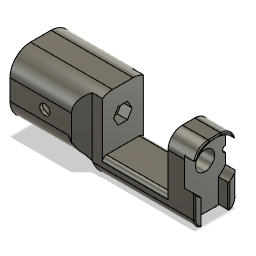
Overall_Assembly2 v12 (Autodesk Fusion 360 archive; units mm, degrees)
design "ElbowFork_4"
Autodesk Fusion 360 part; units mm, degrees
sketch "Sketch1" plane through (0, 0, 0) normal (0, 1, 0) x (1, 0, 0)
  line L0 (-40, 15) -> (-10, 15)
  line L1 (-10, 15) -> (-10, -15)
  line L2 (-40, -15) -> (-10, -15)
  line L3 (-10, -15) -> (-6.6882, -19.9677)
  line L4 (-5, 0) -> (-5, 15)
  line L5 (27, 0) -> (27, 15)
  line L6 (-5, 0) -> (-5, -10)
  line L7 (-5, -10) -> (27, -10)
  line L8 (27, -10) -> (27, 0)
  line L9 (30, -19.9677) -> (-6.6882, -19.9677)
  line L10 (30, 15) -> (40, 15)
  line L11 (40, 15) -> (40, -19.9677)
  line L12 (40, -19.9677) -> (30, -19.9677)
  line L13 (-10, 15) -> (-5, 15)
  line L14 (27, 15) -> (30, 15)
  line L15 (27, 15) -> (30, 15)
  line L16 (-40, 0) -> (-40, 15)
  line L17 (-40, 0) -> (-40, -15)
  constraint perpendicular L1 L2
  constraint perpendicular L4 L13
  constraint coincident L5.end L13
  constraint parallel L4 L6
  constraint perpendicular L4 L7
  constraint perpendicular L7 L8
  constraint collinear L13 L14
  constraint perpendicular L0 L16
  constraint perpendicular L2 L17
extrude "Extrude1" add sketch "Sketch1" along normal blind 30 makes body 1
sketch "Sketch2" plane through (-40, 0, 0) normal (-1, 0, 0) x (0, 0, 1)
  line L0 (-15, 0) -> (15, 0)
  line L1 (15, 0) -> (15, 30)
  line L2 (15, 30) -> (-15, 30)
  line L3 (-15, 30) -> (-15, 0)
  line L4 (-15, 0) -> (15, 0)
  line L5 (15, 0) -> (15, 30)
  line L6 (15, 30) -> (-15, 30)
  line L7 (-15, 30) -> (-15, 0)
  circle A0 centre (0, 15) radius 13.6
  point P0 (0, 15)
  dimension "d37" = 27.2
  constraint coincident P0 A0.centre
  measures "d37" diameter of A0
extrude "Extrude2" cut sketch "Sketch2" against normal blind 22 contours A0 bodies 1
sketch "Sketch3" plane through (0, 30, 0) normal (0, 1, 0) x (-1, 0, 0)
  line L0 (40, -15) -> (40, 15)
  line L1 (40, 15) -> (10, 15)
  line L2 (10, 15) -> (6.6882, 19.9677)
  line L3 (6.6882, 19.9677) -> (-40, 19.9677)
  line L4 (-40, 19.9677) -> (-40, -15)
  line L5 (-40, -15) -> (-27, -15)
  line L6 (-27, -15) -> (-27, 10)
  line L7 (-27, 10) -> (5, 10)
  line L8 (5, 10) -> (5, -15)
  line L9 (5, -15) -> (40, -15)
  line L10 (10, 15) -> (10, -15)
  constraint coincident L1.end L2.start
  constraint coincident L9 L10.end
  constraint perpendicular L9 L10
extrude "Extrude3" cut sketch "Sketch3" against normal blind 5 contours L2 L3 L4 L5 L6 L7 L8 L9 L10 bodies 1
extrude "Extrude4" cut sketch "Sketch1" along normal blind 5 contours L1 L3 L4 L5 L6 L7 L8 L9 L10 L11 L12 L13 L14 L15 bodies 1
chamfer "Chamfer1" distance 5 angle 45 2 edges at (-10, 30, 0) (-10, 0, 0) on bodies 1
fillet "Fillet1" radius 10 4 edges at (-27.5, 30, -15) (-27.5, 30, 15) (-27.5, 0, -15) (-27.5, 0, 15) on bodies 1
sketch "Sketch4" plane through (40, 0, 0) normal (1, 0, 0) x (0, 0, -1)
  line L0 (-19.9677, 5) -> (15, 5)
  line L1 (15, 5) -> (15, 25)
  line L2 (15, 25) -> (-19.9677, 25)
  line L3 (-19.9677, 25) -> (-19.9677, 5)
  line L4 (2.5, 15) -> (2.5, 5) construction
  circle A0 centre (2.5, 5) radius 1.5
  line L5 (-25, 14.9495) -> (-25, 21.4495)
  line L6 (-25, 14.9495) -> (-25, 8.4495)
  line L7 (-25, 21.4495) -> (-7.6195, 21.4495)
  line L8 (-25, 8.4495) -> (-7.5544, 8.4495)
  arc A1 (-7.5544, 8.4495) -> (-7.6195, 21.4495) centre (2.5, 15) ccw
  circle A2 centre (2.5, 15) radius 4.65
  dimension "d38" = 3
  dimension "d39" = 24
  dimension "d40" = 6.5
  dimension "d41" = 6.5
  dimension "d46" = 9.3
  constraint coincident L0 L4.end
  constraint perpendicular L0 L4
  constraint coincident L4.end A0.centre
  constraint perpendicular L5 L7
  constraint perpendicular L6 L8
  constraint concentric A1 A2
  measures "d38" diameter of A0
  measures "d39" diameter of A1
  measures "d40" distance of L5.start L5.end
  measures "d41" distance of L5.start L6.end
  measures "d46" diameter of A2
extrude "Extrude5" cut sketch "Sketch4" against normal blind 5 contours L0 L2 L3 A0 L7 L8 A1 | A2 bodies 1
extrude "Extrude6" cut sketch "Sketch4" against normal blind 16 contours A2 bodies 1
fillet "Fillet2" radius 2 2 edges at (11, 25, 10) (11, 5, 10) on bodies 1
sketch "Sketch5" plane through (-5, 0, 0) normal (1, 0, 0) x (0, 0, -1)
  arc A0 (13.6603, 5) -> (15, 10) centre (5, 10) ccw
  line L0 (15, 10) -> (15, 20)
  arc A1 (15, 20) -> (13.6603, 25) centre (5, 20) ccw
  line L1 (13.6603, 25) -> (-12, 25)
  arc A2 (-10, 23) -> (-12, 25) centre (-12, 23) ccw
  line L2 (-10, 23) -> (-10, 7)
  arc A3 (-12, 5) -> (-10, 7) centre (-12, 7) ccw
  line L3 (-12, 5) -> (13.6603, 5)
  line L4 (4.45, 11.6225) -> (2.5, 10.4967)
  line L5 (-1.4, 15) -> (-1.4, 17.2517)
  line L6 (0.55, 18.3775) -> (-1.4, 17.2517)
  line L7 (4.45, 18.3775) -> (6.4, 17.2517)
  line L8 (4.45, 18.3775) -> (2.5, 19.5033)
  line L9 (0.55, 18.3775) -> (2.5, 19.5033)
  line L10 (0.55, 11.6225) -> (-1.4, 12.7483)
  line L11 (4.45, 11.6225) -> (6.4, 12.7483)
  line L12 (6.4, 15) -> (6.4, 17.2517)
  line L13 (-1.4, 15) -> (-1.4, 12.7483)
  line L14 (0.55, 11.6225) -> (2.5, 10.4967)
  line L15 (6.4, 15) -> (6.4, 12.7483)
  circle A4 centre (2.5, 15) radius 2.5
  dimension "d36" = 5
  measures "d36" diameter of A4
extrude "Extrude9" cut sketch "Sketch5" against normal blind 5 contours L4 L5 L6 L7 L8 L9 L10 L11 L12 L13 L14 L15 | A4 bodies 1
extrude "Extrude8" cut sketch "Sketch5" against normal blind 15 contours A4 bodies 1
fillet "Fillet3" radius 7 2 edges at (33.5, 25, -15) (33.5, 5, -15) on bodies 1
fillet "Fillet4" radius 4.5 2 edges at (16.6559, 25, 19.9677) (16.6559, 5, 19.9677) on bodies 1
sketch "Sketch6" plane through (0, 30, 0) normal (0, 1, 0) x (-1, 0, 0)
  line L0 (40, 5) -> (16.6667, 5)
  line L1 (16.6667, 5) -> (15, 7.5)
  line L2 (15, 7.5) -> (15, -5)
  line L3 (15, -5) -> (40, -5)
  line L4 (40, -5) -> (40, 5)
  circle A0 centre (28, 0) radius 2.5
  dimension "d33" = 5
  measures "d33" diameter of A0
extrude "Extrude10" cut sketch "Sketch6" against normal blind 58 contours A0 bodies 1
copy_body "Body->Comp1" bodies 1 removing the originals makes body 2 in component "Component"
extrude "Extrude1'" cut 1 faces at (40, 5.54, -2.6771) along direction (-1, 0, 0) blind 9 on bodies 2 bodies 2 in component "Component"
fillet "Fillet1'" radius 0.5 14 edges at (40, 25, 9.8005) (40, 24.0016, 18.2941) (40, 5.9661, 18.2536) (40, 5, 9.8005) (40, 22.4594, -13.3958) (40, 15, -15) (40, 7.5406, -13.3958) (40, 21.4495, 13.7429) (40, 8.4495, 13.6989) (37.5, 21.4495, 19.8664) (37.5, 8.4495, 19.8434) (35, 8.9711, 19.9365) (35, 15, 19.9677) (35, 20.9775, 19.9423) on bodies 2 in component "Component"
move_face "OffsetFaces1" offset 5 1 faces at (-40, 4.1882, 10.0012) on bodies 2 in component "Component"
move_face "OffsetFaces2" offset -1 1 faces at (5.6667, 12.3333, 10) on bodies 2 in component "Component"
component "Component" placed x (1, 0, 0) y (0, 1, 0) z (0, 0, 1) at (0, 0, 0)

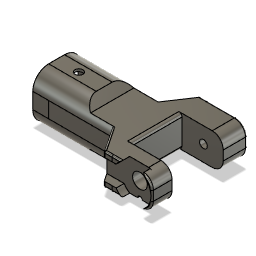
design "SholderFork_1"
Autodesk Fusion 360 part; units mm, degrees
sketch "Sketch1" plane through (0, 0, 0) normal (0, 1, 0) x (1, 0, 0)
  line L0 (-50, -15) -> (-10, -15)
  line L1 (-50, 15) -> (-10, 15)
  line L2 (5, -15) -> (5, 15)
  line L3 (30, 30) -> (5, 30)
  line L4 (30, -30) -> (5, -30)
  line L5 (5, -15) -> (30, -15)
  line L6 (30, -15) -> (30, -30)
  line L7 (5, 15) -> (30, 15)
  line L8 (30, 15) -> (30, 30)
  line L9 (-10, -15) -> (0, -30)
  line L10 (0, -30) -> (5, -30)
  line L11 (-10, 15) -> (0, 30)
  line L12 (0, 30) -> (5, 30)
  line L13 (-10, 15) -> (-10, -15)
  line L14 (-50, 15) -> (-60, 15)
  line L15 (-60, 15) -> (-60, -15)
  line L16 (-60, -15) -> (-50, -15)
  constraint horizontal L3
  constraint perpendicular L2 L5
  constraint perpendicular L4 L6
  constraint perpendicular L2 L7
  constraint perpendicular L3 L8
  constraint perpendicular L0 L13
  constraint perpendicular L14 L15
extrude "Extrude1" add sketch "Sketch1" along normal blind 30 makes body 1
sketch "Sketch3" plane through (-60, 0, 0) normal (-1, 0, 0) x (0, 0, 1)
  line L0 (-15, 0) -> (15, 0)
  line L1 (15, 0) -> (15, 30)
  line L2 (15, 30) -> (-15, 30)
  line L3 (-15, 30) -> (-15, 0)
  circle A0 through (13.6, 15, 10) (-6.8, 26.7779, 10) (-6.8, 3.2221, 10)
  line L4 (-15, 0) -> (15, 0)
  line L5 (15, 0) -> (15, 30)
  line L6 (15, 30) -> (-15, 30)
  line L7 (-15, 30) -> (-15, 0)
  dimension "d64" = 27.2
extrude "Extrude3" cut sketch "Sketch3" against normal blind 36 contours A0 in plane through (-70, 0, 0) normal (-1, 0, 0) bodies 1
sketch "Sketch4" plane through (0, 30, 0) normal (0, 1, 0) x (-1, 0, 0)
  line L0 (50, 15) -> (10, 15)
  line L1 (10, 15) -> (0, 30)
  line L2 (0, 30) -> (-5, 30)
  line L3 (-5, 30) -> (-30, 30)
  line L4 (-30, 30) -> (-30, 15)
  line L5 (-30, 15) -> (-5, 15)
  line L6 (-5, 15) -> (-5, -15)
  line L7 (-5, -15) -> (-30, -15)
  line L8 (-30, -15) -> (-30, -30)
  line L9 (-30, -30) -> (-5, -30)
  line L10 (-5, -30) -> (0, -30)
  line L11 (0, -30) -> (10, -15)
  line L12 (10, -15) -> (60, -15)
  line L13 (25, -10) -> (25, -15)
  line L14 (25, -10) -> (25, 15)
  line L15 (60, -15) -> (60, 15)
  line L16 (60, 15) -> (50, 15)
  constraint coincident L12 L13.end
  constraint perpendicular L12 L13
  constraint coincident L0 L14.end
  constraint perpendicular L0 L14
extrude "Extrude4" cut sketch "Sketch4" against normal blind 5 contours L0 L1 L2 L3 L4 L5 L6 L7 L8 L9 L10 L11 L12 L13 L14 bodies 1
sketch "Sketch5" plane through (0, 0, 0) normal (0, -1, 0) x (1, 0, 0)
  line L0 (-60, -15) -> (-10, -15)
  line L1 (-10, -15) -> (0, -30)
  line L2 (0, -30) -> (5, -30)
  line L3 (5, -30) -> (30, -30)
  line L4 (30, -30) -> (30, -15)
  line L5 (30, -15) -> (5, -15)
  line L6 (5, -15) -> (5, 15)
  line L7 (5, 15) -> (30, 15)
  line L8 (30, 15) -> (30, 30)
  line L9 (30, 30) -> (5, 30)
  line L10 (5, 30) -> (0, 30)
  line L11 (0, 30) -> (-10, 15)
  line L12 (-10, 15) -> (-50, 15)
  line L13 (-25, 14) -> (-25, 15)
  line L14 (-25, 14) -> (-25, -15)
  line L15 (-50, 15) -> (-60, 15)
  line L16 (-60, 15) -> (-60, -15)
  constraint coincident L12 L13.end
  constraint perpendicular L12 L13
  constraint perpendicular L12 L14
extrude "Extrude5" cut sketch "Sketch5" against normal blind 5 contours L0 L1 L2 L3 L4 L5 L6 L7 L8 L9 L10 L11 L12 L13 L14 bodies 1
chamfer "Chamfer1" distance 5 angle 45 2 edges at (-25, 0, 0) (-25, 30, 0) on bodies 1
fillet "Fillet2" radius 10 4 edges at (-45, 30, -15) (-40, 30, 15) (-40, 0, 15) (-45, 0, -15) on bodies 1
sketch "Sketch2" plane through (0, 0, 30) normal (0, 0, 1) x (1, 0, 0)
  line L0 (30, 5) -> (30, 25)
  line L1 (5, 25) -> (5, 5)
  line L2 (5, 5) -> (30, 5)
  line L3 (30, 25) -> (5, 25)
  line L4 (11.0494, 5) -> (23.9506, 5)
  arc A0 (23.9506, 5) -> (23.9506, 25) centre (17.5, 15) ccw
  arc A1 (19, 5) -> (16, 5) centre (17.5, 5) ccw
  line L5 (5.6, 8.5) -> (7.5321, 8.5)
  line L6 (5.6, 21.5) -> (7.5321, 21.5)
  line L7 (5.6, 21.5) -> (5, 21.5)
  line L8 (5.6, 8.5) -> (5, 8.5)
  arc A2 (11.0494, 25) -> (7.5321, 21.5) centre (17.5, 15) ccw
  arc A3 (7.5321, 8.5) -> (11.0494, 5) centre (17.5, 15) ccw
  line L9 (5, 21.5) -> (-2, 21.5)
  line L10 (5, 8.5) -> (-2, 8.5)
  line L11 (-2, 8.5) -> (-4, 8.5)
  line L12 (-4, 8.5) -> (-4, 21.5)
  line L13 (-2, 21.5) -> (-4, 21.5)
  circle A4 centre (17.5, 15) radius 4.65
  dimension "d65" = 23.8
  dimension "d69" = 9.3
  constraint coincident L3 A0.end
  constraint coincident L3 A2.start
  constraint coincident L2 L4.end
  constraint concentric A0 A2
  constraint coincident L2 A1.end
  constraint coincident L2 A1.start
  constraint coincident L5.end A2
  constraint coincident L1 L7.end
  constraint perpendicular L1 L7
  constraint coincident L1 L8.end
  constraint perpendicular L1 L8
  constraint concentric A2 A3
  constraint perpendicular L1 L9
  constraint perpendicular L10 L12
  constraint perpendicular L12 L13
  measures "d65" diameter of A2
  measures "d69" diameter of A4
extrude "Extrude6" cut sketch "Sketch2" against normal blind 5 contours L1 L2 L3 L4 A0 A1 L5 L6 L7 L8 A2 A3 | L1 L9 L10 L11 L12 L13 | A4 bodies 1
copy_body "Body->Comp1" bodies 1 removing the originals makes body 2 in component "Component"
fillet "Fillet2'" radius 2 2 edges at (5, 25, 0) (5, 5, 0) on bodies 2 in component "Component"
extrude "Extrude1'" cut sketch "Sketch2" against normal blind 16 contours A4 bodies 2 in component "Component"
sketch "Sketch6" plane through (0, 0, -30) normal (0, 0, -1) x (-1, 0, 0)
  line L0 (-30, 5) -> (-5, 5)
  line L1 (-5, 5) -> (-5, 25)
  line L2 (-5, 25) -> (-30, 25)
  line L3 (-30, 25) -> (-30, 5)
  circle A0 centre (-17.5, 15) radius 2.45
  point P0 (-17.5, 15)
  dimension "d33" = 4.9
  constraint coincident P0 A0.centre
  measures "d33" diameter of A0
extrude "Extrude5'" cut sketch "Sketch6" against normal blind 16 contours A0 bodies 2 in component "Component"
sketch "Sketch7" plane through (0, 0, -30) normal (0, 0, -1) x (-1, 0, 0)
  circle A0 centre (-17.5, 15) radius 2.45
  line L0 (-30, 5) -> (-5, 5)
  line L1 (-5, 5) -> (-5, 25)
  line L2 (-5, 25) -> (-30, 25)
  line L3 (-30, 25) -> (-30, 5)
  line L4 (-13.6, 15) -> (-13.6, 17.2517)
  line L5 (-13.6, 15) -> (-13.6, 12.7483)
  line L6 (-15.55, 18.3775) -> (-17.5, 19.5033)
  line L7 (-15.55, 18.3775) -> (-13.6, 17.2517)
  line L8 (-19.45, 18.3775) -> (-21.4, 17.2517)
  line L9 (-19.45, 18.3775) -> (-17.5, 19.5033)
  line L10 (-21.4, 15) -> (-21.4, 12.7483)
  line L11 (-21.4, 15) -> (-21.4, 17.2517)
  line L12 (-19.45, 11.6225) -> (-17.5, 10.4967)
  line L13 (-19.45, 11.6225) -> (-21.4, 12.7483)
  line L14 (-15.55, 11.6225) -> (-13.6, 12.7483)
  line L15 (-15.55, 11.6225) -> (-17.5, 10.4967)
  dimension "d40" = 3.9
  measures "d40" distance of A0.centre L4.start
extrude "Extrude6'" cut sketch "Sketch7" against normal blind 5 contours L4 L5 L6 L7 L8 L9 L10 L11 L12 L13 L14 L15 bodies 2 in component "Component"
fillet "Fillet3" radius 7 4 edges at (30, 25, 22.5) (30, 25, -22.5) (30, 5, 22.5) (30, 5, -22.5) on bodies 2 in component "Component"
move_face "OffsetFaces1" offset -2.25 1 faces at (7.6167, 15, 15) on bodies 2 in component "Component"
sketch "Sketch10" plane through (0, 30, 0) normal (0, 1, 0) x (-1, 0, 0)
  line L0 (60, 5) -> (30, 5)
  line L1 (30, -5) -> (60, -5)
  circle A0 centre (46, -0.0923) radius 2.5
  line L2 (30, 5) -> (30, -5)
  line L3 (60, -5) -> (60, 5)
  dimension "d58" = 5
  measures "d58" diameter of A0
extrude "Extrude8" cut sketch "Sketch10" against normal blind 32 contours A0 bodies 2 in component "Component"
fillet "Fillet4" radius 1 21 edges at (2.5, 25, -30) (14, 25, -30) (27.9497, 22.9497, -30) (30, 15, -30) (27.9497, 7.0503, -30) (14, 5, -30) (2.5, 5, -30) (-5.4466, 25, -21.8301) (-5.4466, 5, -21.8301) (8.0247, 25, 30) (2.5, 25, 30) (-5.4466, 25, 21.8301) (2.5, 5, 30) (8.0247, 5, 30) (-5.4466, 5, 21.8301) (0, 6.75, 30) (0, 23.25, 30) (0, 15, -30) (28.3173, 22.5526, 30) (30, 15, 30) (28.3173, 7.4474, 30) on bodies 2 in component "Component"
extrude "Extrude9" cut 1 faces at (17.3887, 5.4875, 30) along direction (0, 0, -1) blind 9 on bodies 2 bodies 2 in component "Component"
move_face "OffsetFaces2" offset -1 1 faces at (5, 17.6667, 6.5) on bodies 2 in component "Component"
component "Component" placed x (1, 0, 0) y (0, 1, 0) z (0, 0, 1) at (0, 0, 0)

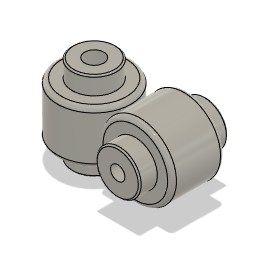
design "ShoulderAxle_1"
Autodesk Fusion 360 part; units mm, degrees
cylinder "CylinderPrimitive1" add diameter 25 height 30 placed x (1, 0, 0) y (0, 0, -1) z (0, 1, 0) at (0, 0, 0) makes body 1
ref_plane "WorkPlane1" through (10, 0, 0) normal (1, 0, 0) x (0, 1, 0)
sketch "Sketch2" plane through (10, 0, 0) normal (1, 0, 0) x (0, 0, -1)
  circle A0 centre (0, 15) radius 6
extrude "Extrude1" add sketch "Sketch2" along normal blind -3 and the other way blind -10 bodies 1
sketch "Sketch3" plane through (0, 0, 0) normal (0, 0, 1) x (1, 0, 0)
  circle A0 centre (23, 15) radius 12.5
  dimension "d27" = 25
  measures "d27" diameter of A0
extrude "Extrude2" add sketch "Sketch3" along normal mid plane 30 bodies 1
sketch "Sketch4" plane through (0, 30, 0) normal (0, 1, 0) x (-1, 0, 0)
  circle A0 centre (0, 0) radius 12.5
  circle A1 centre (0, 0) radius 3.25
  dimension "d10" = 6.5
  constraint concentric A0 A1
  measures "d10" diameter of A1
extrude "Extrude3" cut sketch "Sketch4" against normal blind 16 contours A1 bodies 1
sketch "Sketch5" plane through (0, 0, -15) normal (0, 0, -1) x (-1, 0, 0)
  circle A0 centre (-23, 15) radius 3.25
  circle A1 centre (-23, 15) radius 12.5
  dimension "d13" = 6.5
  measures "d13" diameter of A0
extrude "Extrude4" cut sketch "Sketch5" against normal blind 16 contours A0 bodies 1
copy_body "Body->Comp1" bodies 1 removing the originals makes body 2 in component "Component"
sketch "Sketch8" plane through (0, 0, 1) normal (0, 0, -1) x (-1, 0, 0)
  circle A0 centre (-23, 15) radius 3.25
  line L0 (-17.9794, 13.9286) -> (-20.013, 13.7191)
  line L1 (-17.9794, 13.9286) -> (-20.1526, 13.4333)
  point P0 (-17, 11.75)
  constraint coincident A0 L0.end
  constraint coincident A0 L1.end
extrude "Extrude3'" add sketch "Sketch8" along normal blind 7 contours A0 L0 L1 bodies 2 in component "Component"
sketch "Sketch9" plane through (0, 14, 0) normal (0, 1, 0) x (-1, 0, 0)
  circle A0 centre (0, 0) radius 3.25
  line L0 (2.75, 0) -> (2.75, -1.7321)
  line L1 (2.75, 0) -> (2.75, 1.7321)
  constraint coincident A0 L0.end
  constraint coincident A0 L1.end
extrude "Extrude4'" add sketch "Sketch9" against normal blind 0.5 contours A0 L0 L1 picked at (3.0727, 0.1517) bodies 2 in component "Component"
sketch "Sketch6" plane through (0, 0, 0) normal (0, -1, 0) x (1, 0, 0)
  circle A0 centre (0, 0) radius 12.5
  circle A1 centre (0, 0) radius 2.45
  dimension "d16" = 4.9
  constraint concentric A0 A1
  measures "d16" diameter of A1
extrude "Extrude1'" cut sketch "Sketch6" against normal blind 15 contours A1 bodies 2 in component "Component"
sketch "Sketch7" plane through (0, 0, 15) normal (0, 0, 1) x (1, 0, 0)
  circle A0 centre (23, 15) radius 2.45
  circle A1 centre (23, 15) radius 12.5
  dimension "d19" = 4.9
  measures "d19" diameter of A0
extrude "Extrude2'" cut sketch "Sketch7" against normal blind 20 contours A0 bodies 2 in component "Component"
extrude "Extrude5" cut 1 faces at (-2.9712, 14, -0.1615) along direction (0, -1, 0) blind 7 on bodies 2 bodies 2 in component "Component"
extrude "Extrude6" cut 1 faces at (25.364, 13.1928, 1) along direction (0, 0, 1) blind 7 on bodies 2 bodies 2 in component "Component"
sketch "Sketch12" plane through (0, 0, -15) normal (0, 0, -1) x (-1, 0, 0)
  circle A0 centre (-23, 15) radius 3.25
  circle A1 centre (-23, 15) radius 12.5
  circle A2 centre (-23, 15) radius 7.5
  dimension "d32" = 15
  constraint concentric A0 A2
  measures "d32" diameter of A2
sketch "Sketch13" plane through (0, 0, 15) normal (0, 0, 1) x (1, 0, 0)
  circle A0 centre (23, 15) radius 2.45
  circle A1 centre (23, 15) radius 12.5
  circle A2 centre (23, 15) radius 7.5
  dimension "d33" = 15
  constraint concentric A0 A2
  measures "d33" diameter of A2
extrude "Extrude7" cut sketch "Sketch12" against normal blind 6 contours A1 bodies 2 in component "Component"
extrude "Extrude8" cut sketch "Sketch13" against normal blind 6 contours A1 bodies 2 in component "Component"
sketch "Sketch14" plane through (0, 30, 0) normal (0, 1, 0) x (-1, 0, 0)
  circle A0 centre (0, 0) radius 3.25
  circle A1 centre (0, 0) radius 12.5
  circle A2 centre (0, 0) radius 7.5
  dimension "d38" = 15
  constraint coincident A0.centre A1.centre
  measures "d38" diameter of A2
sketch "Sketch15" plane through (0, 0, 0) normal (0, -1, 0) x (1, 0, 0)
  circle A0 centre (0, 0) radius 2.45
  circle A1 centre (0, 0) radius 12.5
  circle A2 centre (0, 0) radius 7.5
  dimension "d39" = 15
  constraint concentric A0 A2
  measures "d39" diameter of A2
extrude "Extrude9" cut sketch "Sketch14" against normal blind 6 contours A1 bodies 2 in component "Component"
extrude "Extrude10" cut sketch "Sketch15" against normal blind 6 contours A1 bodies 2 in component "Component"
fillet "Fillet1" radius 1.5 4 edges at (-11.6541, 24, -4.5202) (-11.6541, 6, 4.5202) (11.3459, 19.5202, 9) (11.3459, 10.4798, -9) on bodies 2 in component "Component"
fillet "Fillet2" radius 0.5 4 edges at (6.9925, 30, -2.7121) (29.9925, 12.2879, -15) (16.0075, 12.2879, 15) (-6.9925, 0, -2.7121) on bodies 2 in component "Component"
component "Component" placed x (1, 0, 0) y (0, 1, 0) z (0, 0, 1) at (0, 0, 0)

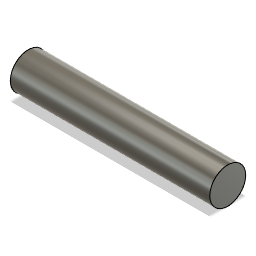
design "Back_connector1"
Autodesk Fusion 360 part; units mm, degrees
sketch "Sketch1" plane through (0, 0, 0) normal (1, 0, 0) x (0, 0, -1)
  circle A0 centre (0, 50) radius 13.5
  dimension "d4" = 27
  measures "d4" diameter of A0
extrude "Extrude1" add sketch "Sketch1" along normal blind 150 makes body 1
copy_body "Body->Comp1" bodies 1 removing the originals makes body 2 in component "Component"
component "Component" placed x (1, 0, 0) y (0, 1, 0) z (0, 0, 1) at (0, 0, 0)

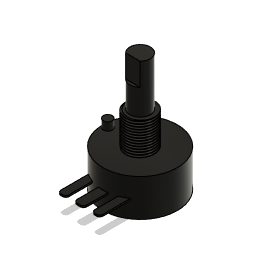
design "potentiometer_basic"
Autodesk Fusion 360 part; units mm, degrees
sketch "Sketch1" plane through (0, 0, 0) normal (0, 1, 0) x (1, 0, 0)
  circle A0 centre (0, 0) radius 11.5
  dimension "d1" = 23
  constraint coincident A0.centre origin
  measures "d1" diameter of A0
extrude "Extrude1" add sketch "Sketch1" along normal blind 11.5 makes body 1
sketch "Sketch2" plane through (0, 11.5, 0) normal (0, 1, 0) x (-1, 0, 0)
  circle A0 centre (0, 0) radius 11.5
  circle A1 centre (0, 0) radius 3.175
  dimension "d4" = 6.35
  constraint coincident A0.centre A1.centre
  measures "d4" diameter of A1
extrude "Extrude2" add sketch "Sketch2" along normal blind 25 contours A1 bodies 1
thread "Thread2" "ISO Metric profile 9.0 M9x0.75 6g" major diameter 8.908 minor diameter 8.0475 pitch 0.75 angle 60 modelled right hand crest width 0.1053 on face at (-3.1592, 19.8333, -0.3161) from (0, 11.5, 0) to (0, 21.5, 0) crest through (-4.454, 11.3125, 0) on bodies 1
sketch "Sketch5" plane through (0, 36.5, 0) normal (0, 1, 0) x (-1, 0, 0)
  circle A0 centre (0, 0) radius 4.454
  circle A1 centre (0, 0) radius 3.175
  dimension "d26" = 6.35
  constraint concentric A0 A1
  measures "d26" diameter of A1
extrude "Extrude4" cut sketch "Sketch5" against normal blind 15 contours A0 | A1 bodies 1
copy_body "Body->Comp1" bodies 1 removing the originals makes body 2 in component "Component"
ref_plane "WorkPlane1" through (0, 0, 13.5) normal (0, 0, 1) x (1, 0, 0)
sketch "Sketch3" plane through (0, 0, 13.5) normal (0, 0, 1) x (1, 0, 0)
  line L0 (0, 5) -> (-6.5, 5)
  line L1 (0, 5) -> (6.5, 5)
  line L2 (-6.5, 5) -> (-6.5, 5.5)
  line L3 (-6.5, 5.5) -> (6.5, 5.5)
  line L4 (6.5, 5.5) -> (6.5, 5)
  dimension "d10" = 6.5
  dimension "d11" = 6.5
  constraint perpendicular L0 L2
  constraint perpendicular L2 L3
  measures "d10" distance of L0.start L0.end
  measures "d11" distance of L0.start L1.end
extrude "Extrude1'" add sketch "Sketch3" against normal blind 6 bodies 2 in component "Component"
move_face "OffsetFaces1" offset 5.5 1 faces at (2.1667, 5.3333, 13.5) on bodies 2 in component "Component"
sketch "Sketch4" plane through (0, 5.5, 0) normal (0, 1, 0) x (-1, 0, 0)
  arc A0 (6.5, 9.4868) -> (-6.5, 9.4868) centre (0, 0) ccw
  line L0 (6.5, 9.4868) -> (6.5, 19)
  line L1 (6.5, 19) -> (-6.5, 19)
  line L2 (-6.5, 19) -> (-6.5, 9.4868)
  line L3 (4, 18.5) -> (4, 10.7819)
  line L4 (-4, 18.5) -> (-4, 10.7819)
  line L5 (1.5, 18.5) -> (1.5, 11.4018)
  line L6 (-1.5, 18.5) -> (-1.5, 11.4018)
  line L7 (-1.5, 18.5) -> (-1.5, 19)
  line L8 (-4, 18.5) -> (-4, 19)
  line L9 (1.5, 18.5) -> (1.5, 19)
  line L10 (4, 18.5) -> (4, 19)
  constraint coincident A0 L3.end
  constraint perpendicular L1 L3
  constraint coincident A0 L4.end
  constraint perpendicular L1 L4
  constraint coincident A0 L5.end
  constraint parallel L3 L5
  constraint coincident A0 L6.end
  constraint perpendicular L1 L6
  constraint coincident L1 L7.end
  constraint perpendicular L1 L7
  constraint coincident L1 L8.end
  constraint perpendicular L1 L8
  constraint coincident L1 L9.end
  constraint parallel L5 L9
  constraint coincident L1 L10.end
  constraint perpendicular L1 L10
extrude "Extrude2'" cut sketch "Sketch4" against normal blind 7 contours A0 L1 L3 L5 L9 L10 | A0 L1 L4 L6 L7 L8 bodies 2 in component "Component"
fillet "Fillet1" radius 1 6 edges at (-4, 5.25, 19) (-1.5, 5.25, 19) (1.5, 5.25, 19) (4, 5.25, 19) (6.5, 5.25, 19) (-6.5, 5.25, 19) on bodies 2 in component "Component"
sketch "Sketch7" plane through (0, 21.5, 0) normal (0, 1, 0) x (-1, 0, 0)
  spline S0 degree 3 poles (-2.5371, -3.6608) (-2.2066, -3.8678) (-1.8503, -4.0305) (-1.1087, -4.2562) (-0.7271, -4.3195) (0.2177, -4.349) (0.7755, -4.258) (1.8144, -3.8692) (2.2869, -3.5788) (3.0851, -2.8388) (3.4058, -2.3994) (3.8545, -1.4308) (3.9818, -0.9127) (4.0053, -0.3849) knots -0.884633 -0.884633 -0.884633 -0.884633 -0.767855 -0.767855 -0.652496 -0.652496 -0.484765 -0.484765 -0.320104 -0.320104 -0.158516 -0.158516 0 0 0 0
  arc A0 (4.0053, -0.3849) -> (1.6693, 3.6611) centre (0, 0) ccw
  spline S1 degree 3 poles (1.6693, 3.6611) (1.3528, 3.8256) (1.0158, 3.9471) (0.3141, 4.1004) (-0.0478, 4.1302) (-0.9508, 4.0858) (-1.4822, 3.9526) (-2.4745, 3.4872) (-2.9241, 3.156) (-3.6795, 2.3333) (-3.9752, 1.8471) (-4.369, 0.7796) (-4.4596, 0.2071) (-4.4389, -0.3668) knots -0.886518 -0.886518 -0.886518 -0.886518 -0.779309 -0.779309 -0.670676 -0.670676 -0.507623 -0.507623 -0.341492 -0.341492 -0.172284 -0.172284 0 0 0 0
  arc A1 (-4.4389, -0.3668) -> (-2.5371, -3.6608) centre (0, 0) ccw
  circle A2 centre (0, 0) radius 3.175
  dimension "d29" = 6.35
  constraint coincident A0.centre A1.centre
  measures "d29" diameter of A2
extrude "Extrude5" add sketch "Sketch7" along normal blind 15 contours A2 bodies 2 in component "Component"
sketch "Sketch8" plane through (0, 36.5, 0) normal (0, 1, 0) x (-1, 0, 0)
  circle A0 centre (0, 0) radius 3.175
  line L0 (0, 3.15) -> (0, 3.175)
  line L1 (0, 2.25) -> (2.2401, 2.25)
  line L2 (0, 2.25) -> (-2.2401, 2.25)
  dimension "d32" = 0.9
  constraint coincident A0 L0.end
  constraint vertical L0
  constraint coincident A0 L1.end
  constraint coincident A0 L2.end
  measures "d32" distance of L0.start L1.start
extrude "Extrude6" cut sketch "Sketch8" against normal blind 7 contours A0 L1 L2 picked at (0.1378, 2.8577) bodies 2 in component "Component"
sketch "Sketch9" plane through (0, 11.5, 0) normal (0, 1, 0) x (-1, 0, 0)
  arc A0 (1.9018, 4.0276) -> (-1.9018, 4.0276) centre (0, 0) ccw
  spline S0 degree 3 poles (1.9018, 4.0276) (2.2464, 3.8449) (2.5654, 3.6177) (3.1317, 3.0883) (3.3772, 2.7894) (3.8752, 1.986) (4.0753, 1.4574) (4.258, 0.3632) (4.2428, -0.1911) (4.001, -1.2524) (3.7808, -1.7498) (3.1663, -2.6227) (2.7814, -2.992) (2.336, -3.2763) knots -0.884633 -0.884633 -0.884633 -0.884633 -0.767855 -0.767855 -0.652496 -0.652496 -0.484765 -0.484765 -0.320104 -0.320104 -0.158516 -0.158516 0 0 0 0
  arc A1 (-2.336, -3.2763) -> (2.336, -3.2763) centre (0, 0) ccw
  spline S1 degree 3 poles (-2.336, -3.2763) (-2.6366, -3.0843) (-2.9104, -2.8533) (-3.394, -2.3222) (-3.6007, -2.0237) (-4.0138, -1.2194) (-4.1642, -0.6926) (-4.2573, 0.3994) (-4.1952, 0.9543) (-3.8604, 2.0199) (-3.5872, 2.519) (-2.8596, 3.3938) (-2.4092, 3.7585) (-1.9018, 4.0276) knots -0.886518 -0.886518 -0.886518 -0.886518 -0.779309 -0.779309 -0.670676 -0.670676 -0.507623 -0.507623 -0.341492 -0.341492 -0.172284 -0.172284 0 0 0 0
  circle A2 centre (0, 0) radius 11.5
  circle A3 centre (10, 0) radius 1.4
  dimension "d35" = 10
  dimension "d36" = 2.8
  measures "d35" distance of A0.centre A3.centre
  measures "d36" diameter of A3
extrude "Extrude7" add sketch "Sketch9" along normal blind 2.5 contours A3 bodies 2 in component "Component"
component "Component" placed x (1, 0, 0) y (0, 1, 0) z (0, 0, 1) at (0, 0, 0)

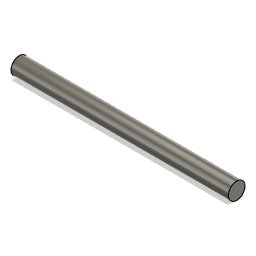
design "Shoulder_connector1"
Autodesk Fusion 360 part; units mm, degrees
sketch "Sketch1" plane through (0, 0, 0) normal (1, 0, 0) x (0, 0, -1)
  circle A0 centre (0, 50) radius 13.5
  dimension "d4" = 27
  measures "d4" diameter of A0
extrude "Extrude1" add sketch "Sketch1" along normal blind 350 makes body 1
copy_body "Body->Comp1" bodies 1 removing the originals makes body 2 in component "Component"
component "Component" placed x (1, 0, 0) y (0, 1, 0) z (0, 0, 1) at (0, 0, 0)

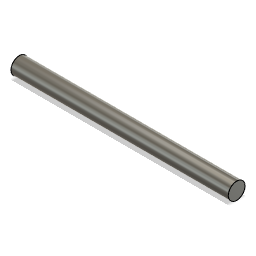
design "Elbow_connector1"
Autodesk Fusion 360 part; units mm, degrees
sketch "Sketch1" plane through (0, 0, 0) normal (1, 0, 0) x (0, 0, -1)
  circle A0 centre (0, 50) radius 13.5
  dimension "d4" = 27
  measures "d4" diameter of A0
extrude "Extrude1" add sketch "Sketch1" along normal blind 350 makes body 1
copy_body "Body->Comp1" bodies 1 removing the originals makes body 2 in component "Component"
component "Component" placed x (1, 0, 0) y (0, 1, 0) z (0, 0, 1) at (0, 0, 0)
